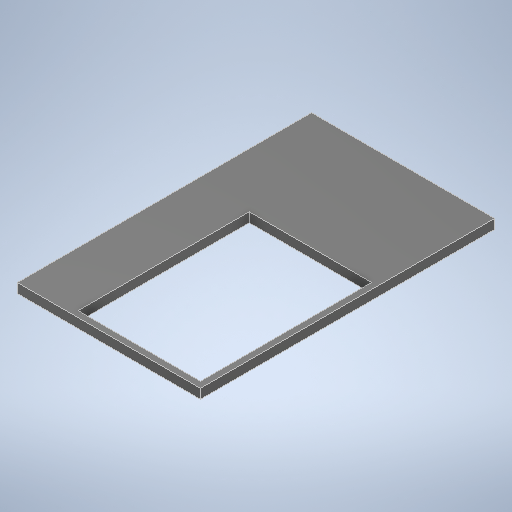
# Autodesk Inventor part: lid
Saved by Autodesk Inventor 2025.2 (Build 292293000, 293)
## iProperties
Created: 2025-08-16
Part Number: lid
Material: Acetal Resin, Black
Document SubType Name: Modeling
Designer: pakiyan
Density: 1.425 g/cm^3
Appearance: Smooth - Black
Author: pakiyan
Autodesk Inventor part; units mm, degrees
ref_plane "YZ Plane" through (0, 0, 0) normal (1, 0, 0) x (0, 1, 0)
ref_plane "XZ Plane" through (0, 0, 0) normal (0, 1, 0) x (-1, 0, 0)
ref_plane "XY Plane" through (0, 0, 0) normal (0, 0, 1) x (1, 0, 0)
sketch "Sketch2" plane through (0, 0, 0) normal (0, 1, 0) x (-1, 0, 0)
  line L0 (37.5, 59.5) -> (-37.5, 59.5)
  line L1 (-37.5, 59.5) -> (-37.5, -59.5)
  line L2 (-37.5, -59.5) -> (37.5, -59.5)
  line L3 (37.5, -59.5) -> (37.5, 59.5)
  line L4 (37.5, 59.5) -> (-37.5, -59.5) construction
  line L5 (-37.5, 59.5) -> (37.5, -59.5) construction
  line L6 (-35, 58.5) -> (15.1, 58.5)
  line L7 (15.1, 58.5) -> (15.1, -11.6)
  line L8 (15.1, -11.6) -> (-35, -11.6)
  line L9 (-35, -11.6) -> (-35, 58.5)
  line L10 (-37.5, 59.5) -> (37.5, 59.5)
  line L11 (37.5, 59.5) -> (37.5, 61)
  line L12 (37.5, 61) -> (-37.5, 61)
  line L13 (-37.5, 61) -> (-37.5, 59.5)
  point P0 (0, 0)
  dimension "d8" = 119
  dimension "d9" = 75
  dimension "d10" = 2.5
  dimension "d11" = 1
  dimension "d12" = 70.1
  dimension "d13" = 50.1
  dimension "d14" = 1.5
  constraints: 28 end point, 6 parallel, 3 horizontal, 3 perpendicular, 2 midpoint
  measures "d8" distance of L0.end L1.end
  measures "d9" distance of L1.end L2.end
  measures "d10" distance between parallel lines of L1 L9
  measures "d11" distance between parallel lines of L0 L6
  measures "d12" distance of L8.end L6.start
  measures "d13" distance of L7.end L8.end
  measures "d14" distance of L12.end L0.end
extrude "Extrusion2" add sketch "Sketch2" along normal blind 3.9
body "Solid2"
